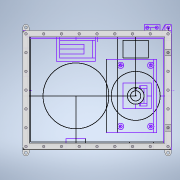
# Autodesk Inventor part: deadbolt enclosure walls
Saved by Autodesk Inventor 2022 (Build 260153000, 153)
## iProperties
Created: 2021-11-30
Part Number: deadbolt enclosure walls
Material: Generic
Document SubType Name: Modeling
Designer: a-dubs
Density: 1 g/cm^3
Appearance: Default
Author: a-dubs
Autodesk Inventor part; units mm, degrees
ref_plane "YZ Plane" through (0, 0, 0) normal (1, 0, 0) x (0, 1, 0)
sketch "Sketch1" plane through (0, 0, 0) normal (0, 1, 0) x (-1, 0, 0)
  line L0 (0, 0) -> (61, 0)
  circle A0 centre (0, 0) radius 33.6
  circle A1 centre (61, 0) radius 8.5
  line L1 (69.5, 0) -> (69.5, 7.5)
  line L2 (69.5, 7.5) -> (69.5, -7.5)
  line L3 (69.5, -7.5) -> (65, -7.5)
  line L4 (69.5, 7.5) -> (65, 7.5)
  line L5 (69.5, 7.5) -> (72.5, 7.5)
  line L6 (72.5, 7.5) -> (72.5, -7.5)
  line L7 (72.5, -7.5) -> (69.5, -7.5)
  line L8 (52.5, 0) -> (47.5, 0)
  line L9 (61, 8.5) -> (61, 13.5)
  line L10 (72.5, 0) -> (77.5, 0)
  line L11 (61, -8.5) -> (61, -13.5)
  line L12 (47.95, 13.05) -> (77.05, 13.05)
  line L13 (77.05, 13.05) -> (77.05, -13.05)
  line L14 (77.05, -13.05) -> (47.95, -13.05)
  line L15 (47.95, -13.05) -> (47.95, 13.05)
  line L16 (72.5, 7.5) -> (72.5, 10.5)
  line L17 (72.5, 10.5) -> (65, 10.5)
  line L18 (65, 10.5) -> (65, 7.5)
  line L19 (72.5, -7.5) -> (72.5, -10.5)
  line L20 (72.5, -10.5) -> (65, -10.5)
  line L21 (65, -10.5) -> (65, -7.5)
  line L22 (61, 0) -> (61, 60)
  line L23 (0, 0) -> (-42.65, 0)
  line L24 (-42.65, 0) -> (-47.65, 0)
  line L25 (0, 0) -> (0, -33.6)
  line L26 (0, 0) -> (42.65, 0)
  line L27 (42.65, 0) -> (42.65, 60)
  line L28 (42.65, 0) -> (42.65, -33.6)
  circle A2 centre (61, 0) radius 25
  line L29 (42.65, 25) -> (42.65, 31.2)
  line L30 (42.65, 31.2) -> (48.85, 31.2)
  line L31 (42.65, -25) -> (42.65, -31.2)
  line L32 (36, 0) -> (31, 0)
  line L33 (31, 0) -> (31, -31.2)
  line L34 (31, -31.2) -> (31, -37.4)
  line L35 (31, -37.4) -> (79.35, -37.4)
  line L36 (79.35, -37.4) -> (79.35, 31.2)
  line L37 (79.35, 31.2) -> (79.35, 37.4)
  line L38 (79.35, 37.4) -> (31, 37.4)
  line L39 (31, 37.4) -> (31, 0)
  line L40 (42.65, -33.6) -> (42.65, -37.4)
  circle A3 centre (61, 0) radius 5.25
  line L41 (86, 0) -> (91, 0)
  line L42 (91, 0) -> (97.4, 0)
  line L43 (-47.65, 0) -> (-47.65, 60)
  line L44 (-47.65, 60) -> (42.65, 60)
  line L45 (91, 0) -> (91, 60)
  line L46 (91, 60) -> (42.65, 60)
  line L47 (0, -33.6) -> (0, -43.6)
  line L48 (0, -43.6) -> (0, -48.6)
  line L49 (0, -48.6) -> (0, -55)
  line L50 (0, -55) -> (-54.05, -55)
  line L51 (0, -48.6) -> (-47.65, -48.6)
  line L52 (-47.65, -48.6) -> (-47.65, 0)
  line L53 (0, -55) -> (97.4, -55)
  line L54 (97.4, -55) -> (97.4, 0)
  line L55 (91, 0) -> (91, -48.6)
  line L56 (91, -48.6) -> (0, -48.6)
  line L57 (0, -48.6) -> (10, -48.6)
  line L58 (0, -48.6) -> (-10, -48.6)
  line L59 (10, -48.6) -> (10, -55)
  line L60 (-10, -48.6) -> (-10, -55)
  line L61 (10, -48.6) -> (10, -43.6)
  line L62 (10, -43.6) -> (-10, -43.6)
  line L63 (-10, -43.6) -> (-10, -49.0563)
  line L64 (65, 10.5) -> (66, 10.5)
  line L65 (66, 10.5) -> (66, 7.5)
  line L66 (65, -10.5) -> (66, -10.5)
  line L67 (66, -10.5) -> (66, -7.5)
  line L68 (-47.65, 0) -> (-54.05, 0)
  line L69 (42.65, 60) -> (42.65, 66.4)
  line L70 (-54.05, -55) -> (-54.05, 0)
  line L71 (-54.05, 66.4) -> (-54.05, 0)
  line L72 (42.65, 66.4) -> (-54.05, 66.4)
  line L73 (97.4, 0) -> (97.4, 66.4)
  line L74 (97.4, 66.4) -> (42.65, 66.4)
  line L75 (-47.65, 60) -> (-50.85, 60)
  line L76 (-50.85, 60) -> (-50.85, 63.2)
  circle A4 centre (-50.85, 63.2) radius 1.6
  line L77 (91, 60) -> (94.2, 60)
  line L78 (94.2, 60) -> (-50.85, 60)
  circle A5 centre (-32.7188, 63.2) radius 1.6
  circle A6 centre (-14.5875, 63.2) radius 1.6
  circle A7 centre (3.5437, 63.2) radius 1.6
  circle A8 centre (21.675, 63.2) radius 1.6
  circle A9 centre (39.8062, 63.2) radius 1.6
  circle A10 centre (57.9375, 63.2) radius 1.6
  circle A11 centre (76.0687, 63.2) radius 1.6
  circle A12 centre (94.2, 63.2) radius 1.6
  line L79 (-47.65, 60) -> (-47.65, 63.2)
  line L80 (-47.65, 63.2) -> (-47.65, -51.8)
  circle A13 centre (-50.85, 44.0333) radius 1.6
  circle A14 centre (-50.85, 24.8667) radius 1.6
  circle A15 centre (-50.85, 5.7) radius 1.6
  circle A16 centre (-50.85, -13.4667) radius 1.6
  circle A17 centre (-50.85, -32.6333) radius 1.6
  circle A18 centre (-50.85, -51.8) radius 1.6
  line L81 (-47.65, 60) -> (21.675, 60)
  line L82 (21.675, 60) -> (21.675, 55.1722)
  line L83 (-47.65, 5.7) -> (-45.15, 5.7)
  circle A19 centre (-32.7188, -51.8) radius 1.6
  circle A20 centre (-14.5875, -51.8) radius 1.6
  circle A21 centre (3.5437, -51.8) radius 1.6
  circle A22 centre (21.675, -51.8) radius 1.6
  circle A23 centre (39.8062, -51.8) radius 1.6
  circle A24 centre (57.9375, -51.8) radius 1.6
  circle A25 centre (76.0687, -51.8) radius 1.6
  circle A26 centre (94.2, -51.8) radius 1.6
  circle A27 centre (94.2, 44.0333) radius 1.6
  circle A28 centre (94.2, 24.8667) radius 1.6
  circle A29 centre (94.2, 5.7) radius 1.6
  circle A30 centre (94.2, -13.4667) radius 1.6
  circle A31 centre (94.2, -32.6333) radius 1.6
  line L84 (61, 60) -> (61, 56.8)
  line L85 (61, 56.8) -> (61, 38.8)
  line L86 (61, 56.8) -> (48.1, 56.8)
  line L87 (61, 56.8) -> (73.9, 56.8)
  line L88 (73.9, 56.8) -> (73.9, 38.8)
  line L89 (73.9, 38.8) -> (61, 38.8)
  line L90 (48.1, 56.8) -> (48.1, 38.8)
  line L91 (48.1, 38.8) -> (61, 38.8)
  line L92 (0, 60) -> (0, 56.8)
  line L93 (0, 56.8) -> (-16.65, 56.8)
  line L94 (-16.65, 56.8) -> (16.65, 56.8)
  line L95 (16.65, 56.8) -> (16.65, 38.6)
  line L96 (16.65, 38.6) -> (-16.65, 38.6)
  line L97 (-16.65, 38.6) -> (-16.65, 56.8)
  circle A32 centre (-50.85, 63.2) radius 1.4
  circle A33 centre (-32.7188, 63.2) radius 1.4
  circle A34 centre (-14.5875, 63.2) radius 1.4
  circle A35 centre (3.5437, 63.2) radius 1.4
  circle A36 centre (21.675, 63.2) radius 1.4
  circle A37 centre (39.8062, 63.2) radius 1.4
  circle A38 centre (57.9375, 63.2) radius 1.4
  circle A39 centre (76.0687, 63.2) radius 1.4
  circle A40 centre (94.2, 63.2) radius 1.4
  circle A41 centre (-50.85, -51.8) radius 1.4
  circle A42 centre (-32.7188, -51.8) radius 1.4
  circle A43 centre (-14.5875, -51.8) radius 1.4
  circle A44 centre (3.5437, -51.8) radius 1.4
  circle A45 centre (21.675, -51.8) radius 1.4
  circle A46 centre (39.8062, -51.8) radius 1.4
  circle A47 centre (57.9375, -51.8) radius 1.4
  circle A48 centre (76.0687, -51.8) radius 1.4
  circle A49 centre (94.2, -51.8) radius 1.4
  circle A50 centre (-50.85, 44.0333) radius 1.4
  circle A51 centre (-50.85, 24.8667) radius 1.4
  circle A52 centre (-50.85, 5.7) radius 1.4
  circle A53 centre (-50.85, -13.4667) radius 1.4
  circle A54 centre (-50.85, -32.6333) radius 1.4
  circle A55 centre (-50.85, -51.8) radius 1.4
  circle A56 centre (94.2, 63.2) radius 1.4
  circle A57 centre (94.2, 44.0333) radius 1.4
  circle A58 centre (94.2, 24.8667) radius 1.4
  circle A59 centre (94.2, 5.7) radius 1.4
  circle A60 centre (94.2, -13.4667) radius 1.4
  circle A61 centre (94.2, -32.6333) radius 1.4
  circle A62 centre (94.2, -51.8) radius 1.4
  line L98 (61, 8.5) -> (61, 6.7)
  line L99 (61, 6.7) -> (61.8, 6.7)
  line L100 (61, 6.7) -> (60.2, 6.7)
  line L101 (60.2, 6.7) -> (60.2, 8.4623)
  line L102 (61.8, 6.7) -> (61.8, 8.4623)
  line L103 (-16.65, 56.8) -> (-16.65, 60)
  line L104 (-16.65, 60) -> (-19.85, 60)
  line L105 (16.65, 38.6) -> (19.85, 38.6)
  line L106 (19.85, 38.6) -> (19.85, 35.4)
  line L107 (-19.85, 60) -> (19.85, 60)
  line L108 (19.85, 60) -> (19.85, 35.4)
  line L109 (19.85, 35.4) -> (-19.85, 35.4)
  line L110 (-19.85, 35.4) -> (-19.85, 60)
  line L111 (-16.65, 47.7) -> (8.35, 47.7)
  line L112 (16.65, 56.8) -> (19.85, 56.8)
  line L113 (16.65, 38.6) -> (19.85, 38.6)
  line L114 (8.35, 47.7) -> (8.35, 52.7)
  line L115 (8.35, 47.7) -> (8.35, 42.7)
  line L116 (8.35, 42.7) -> (-16.65, 42.7)
  line L117 (8.35, 52.7) -> (-16.65, 52.7)
  line L118 (79.35, -37.4) -> (82.55, -37.4)
  line L119 (82.55, -37.4) -> (82.55, 37.4)
  line L120 (82.55, 37.4) -> (79.35, 37.4)
  line L121 (48.85, 31.2) -> (45.65, 31.2)
  circle A63 centre (45.65, 31.2) radius 1.6
  circle A64 centre (45.65, 31.2) radius 1.4
  circle A65 centre (45.65, 31.2) radius 3.2
  circle A66 centre (76.35, 31.2) radius 1.6
  circle A67 centre (76.35, 31.2) radius 1.4
  circle A68 centre (76.35, 31.2) radius 3.2
  circle A69 centre (45.65, -31.2) radius 1.6
  circle A70 centre (45.65, -31.2) radius 1.4
  circle A71 centre (45.65, -31.2) radius 3.2
  circle A72 centre (76.35, -31.2) radius 3.2
  circle A73 centre (76.35, -31.2) radius 1.6
  circle A74 centre (76.35, -31.2) radius 1.4
  line L122 (91, -48.6) -> (92.6, -48.6)
  line L123 (92.6, -48.6) -> (92.6, -50.2)
  line L124 (-47.65, 60) -> (-49.25, 60)
  line L125 (-49.25, 60) -> (-49.25, 61.6)
  line L126 (-47.65, 60) -> (-46.05, 60)
  line L127 (-46.05, 60) -> (-46.05, 58.4)
  line L128 (91, -48.6) -> (89.4, -48.6)
  line L129 (89.4, -48.6) -> (89.4, -47)
  line L130 (89.4, -47) -> (-46.05, -47)
  line L131 (-46.05, -47) -> (-46.05, 58.4)
  line L132 (-46.05, 58.4) -> (89.4, 58.4)
  line L133 (89.4, 58.4) -> (89.4, -47)
  line L134 (-49.25, 61.6) -> (92.6, 61.6)
  line L135 (92.6, 61.6) -> (92.6, -50.2)
  line L136 (92.6, -50.2) -> (-49.25, -50.2)
  line L137 (-49.25, -50.2) -> (-49.25, 61.6)
  line L138 (76.0688, 66.4) -> (69.6688, 66.4)
  line L139 (76.0688, 66.4) -> (76.0688, 69.6)
  line L140 (76.0688, 69.6) -> (80.8688, 69.6)
  line L141 (76.0688, 69.6) -> (72.8688, 69.6)
  line L142 (80.8688, 69.6) -> (82.4688, 69.6)
  circle A75 centre (82.4688, 69.6) radius 1.6
  circle A76 centre (72.8688, 69.6) radius 1.6
  line L143 (69.6688, 66.4) -> (69.6688, 72.8)
  line L144 (76.0688, 66.4) -> (82.4688, 66.4)
  line L145 (82.4688, 66.4) -> (85.6688, 66.4)
  line L146 (85.6688, 66.4) -> (85.6688, 72.8)
  line L147 (85.6688, 72.8) -> (69.6688, 72.8)
  line L148 (57.9375, -51.8) -> (54.6375, -51.8)
  line L149 (54.6375, -51.8) -> (54.6375, -55)
  line L150 (54.6375, -51.8) -> (54.6375, -47)
  line L151 (76.0687, -51.8) -> (79.3687, -51.8)
  line L152 (79.3687, -51.8) -> (79.3688, -47)
  line L153 (79.3687, -51.8) -> (79.3688, -55)
  line L154 (-50.85, 44.0333) -> (-50.85, 48.8333)
  line L155 (-50.85, 24.8667) -> (-50.85, 20.0667)
  line L156 (-50.85, 48.8333) -> (-54.05, 48.8333)
  line L157 (-50.85, 48.8333) -> (-47.65, 48.8333)
  line L158 (-50.85, 20.0667) -> (-47.65, 20.0667)
  line L159 (-50.85, 20.0667) -> (-54.05, 20.0667)
  line L160 (94.2, 44.0333) -> (94.2, 47.4333)
  line L161 (94.2, 44.0333) -> (94.2, 40.6333)
  line L162 (94.2, -32.6333) -> (94.2, -29.2333)
  line L163 (94.2, -32.6333) -> (94.2, -36.0333)
  line L164 (94.2, -36.0333) -> (97.4, -36.0333)
  line L165 (94.2, -36.0333) -> (91, -36.0333)
  line L166 (94.2, -29.2333) -> (91, -29.2333)
  line L167 (94.2, -29.2333) -> (97.4, -29.2333)
  line L168 (94.2, 40.6333) -> (97.4, 40.6333)
  line L169 (94.2, 40.6333) -> (91, 40.6333)
  line L170 (94.2, 47.4333) -> (97.4, 47.4333)
  line L171 (94.2, 47.4333) -> (91, 47.4333)
  line L172 (97.4, 47.4333) -> (97.4, 55.4333)
  line L173 (94.2, 5.7) -> (97.4, 5.7)
  line L174 (97.4, 5.7) -> (97.4, 54.7)
  line L175 (97.4, 54.7) -> (97.4, 58.3)
  line L176 (97.4, 58.3) -> (91, 58.3)
  line L177 (97.4, 66.4) -> (97.4, 56.8)
  line L178 (97.4, 66.4) -> (87.8, 66.4)
  line L179 (87.8, 66.4) -> (87.8, 60)
  line L180 (97.4, 56.8) -> (91, 56.8)
  line L181 (94.2, 63.2) -> (94.2, 69.6)
  circle A77 centre (94.2, 69.6) radius 1.6
  line L182 (97.4, 66.4) -> (91, 66.4)
  line L183 (91, 66.4) -> (91, 72.8)
  line L184 (91, 72.8) -> (97.4, 72.8)
  line L185 (97.4, 72.8) -> (97.4, 66.4)
  line L186 (91, 72.8) -> (87.8, 66.4)
  line L187 (97.4, -55) -> (97.4, 66.4)
  line L188 (97.4, 66.4) -> (97.4, 5.7)
  line L189 (-50.85, 66.4) -> (-50.85, 63.2)
  point P0 (42.65, 37.4)
  point P1 (31, -12.9599)
  point P2 (31, 12.9599)
  point P3 (79.3688, -48.6)
  point P4 (54.6375, -48.6)
  dimension "d1" = 67.2
  dimension "d2" = 17
  dimension "d0" = 61
  dimension "d3" = 7.5
  dimension "d4" = 15
  dimension "d5" = 3
  dimension "d6" = 5
  dimension "d7" = 5
  dimension "d8" = 5
  dimension "d9" = 5
  dimension "d10" = 3
  dimension "d11" = 60
  dimension "d13" = 42.65
  dimension "d14" = 5
  dimension "d16" = 50
  dimension "d17" = 6.2
  dimension "d18" = 6.2
  dimension "d19" = 6.2
  dimension "d26" = 5
  dimension "d27" = 6.2
  dimension "d31" = 10.5
  dimension "d33" = 5
  dimension "d34" = 6.4
  dimension "d36" = 10
  dimension "d37" = 5
  dimension "d38" = 6.4
  dimension "d41" = 10
  dimension "d42" = 10
  dimension "d52" = 1
  dimension "d53" = 1
  dimension "d56" = 6.4
  dimension "d57" = 6.4
  dimension "d58" = 3.2
  dimension "d59" = 3.2
  dimension "d62" = 18.1313
  dimension "d67" = 115
  dimension "d70" = 19.1667
  dimension "d78" = 3.2
  dimension "d79" = 18
  dimension "d80" = 12.9
  dimension "d81" = 12.9
  dimension "d82" = 3.2
  dimension "d83" = 16.65
  dimension "d84" = 33.3
  dimension "d85" = 18.2
  dimension "d93" = 2.8
  dimension "d96" = 18.1313
  dimension "d99" = 115
  dimension "d104" = 19.1667
  dimension "d107" = 145.05
  dimension "d110" = 1.8
  dimension "d111" = 0.8
  dimension "d112" = 0.8
  dimension "d115" = 3.2
  dimension "d116" = 3.2
  dimension "d117" = 3.2
  dimension "d118" = 3.2
  dimension "d119" = 25
  dimension "d120" = 5
  dimension "d121" = 5
  dimension "d127" = 3.2
  dimension "d128" = 3.2
  dimension "d129" = 2.8
  dimension "d130" = 6.4
  dimension "d137" = 1.6
  dimension "d138" = 1.6
  constraints: 380 end point, 83 point on line, 75 centre point, 58 perpendicular, 33 vertical, 28 horizontal, 25 symmetric about line, 20 coincident, 16 parallel, 5 collinear, 5 midpoint, 2 point on circle, 1 horizontal alignment, 125 other
  measures "d0" distance of L0.start L0.end
  measures "d3" distance of L1.start L1.end
  measures "d4" distance of L1.end L2.end
  measures "d5" distance of L1.end L5.end
  measures "d6" distance of L8.start L8.end
  measures "d7" distance of L9.start L9.end
  measures "d8" distance of L10.start L10.end
  measures "d9" distance of L11.start L11.end
  measures "d10" distance of L5.end L16.end
  measures "d11" distance of L22.start L22.end
  measures "d13" distance of L23.start L23.end
  measures "d14" distance of L23.end L24.end
  measures "d16" diameter of A2
  measures "d17" distance of L29.start L29.end
  measures "d18" distance of L29.end L30.end
  measures "d19" distance of L31.start L31.end
  measures "d26" distance of L32.start L32.end
  measures "d27" distance of L33.end L34.end
  measures "d31" diameter of A3
  measures "d33" distance of L41.start L41.end
  measures "d34" distance of L41.end L42.end
  measures "d36" distance of L25.end L47.end
  measures "d37" distance of L47.end L48.end
  measures "d38" distance of L48.end L49.end
  measures "d41" distance of L48.end L57.end
  measures "d42" distance of L48.end L58.end
  measures "d52" distance of L17.end L64.end
  measures "d53" distance of L20.end L66.end
  measures "d56" distance of L24.end L68.end
  measures "d57" distance of L27.end L69.end
  measures "d58" distance of L43.end L75.end
  measures "d59" diameter of A4
  measures "d62" distance of A4.centre A5.centre
  measures "d67" distance of L79.end L80.end
  measures "d70" distance of A4.centre A13.centre
  measures "d78" distance of L22.end L84.end
  measures "d79" distance of L84.end L85.end
  measures "d80" distance of L84.end L86.end
  measures "d81" distance of L84.end L87.end
  measures "d82" distance of L92.start L92.end
  measures "d83" distance of L92.end L93.end
  measures "d84" distance of L93.end L94.end
  measures "d85" distance of L94.end L95.end
  measures "d93" diameter of A32
  measures "d96" distance of A32.centre A33.centre
  measures "d99" distance of A32.centre A41.centre
  measures "d104" distance of A32.centre L154.start
  measures "d107" distance of A32.centre L181.start
  measures "d110" distance of L9.start L98.end
  measures "d111" distance of L98.end L99.end
  measures "d112" distance of L98.end L100.end
  measures "d115" distance of L93.end L103.end
  measures "d116" distance of L103.end L104.end
  measures "d117" distance of L95.end L105.end
  measures "d118" distance of L105.end L106.end
  measures "d119" distance of L111.start L111.end
  measures "d120" distance of L111.end L114.end
  measures "d121" distance of L111.end L115.end
  measures "d127" distance of L121.start L121.end
  measures "d128" diameter of A63
  measures "d129" diameter of A64
  measures "d130" diameter of A65
  measures "d137" distance of L122.end L123.end
  measures "d138" distance of L43.end L124.end
extrude "Extrusion13" add sketch "Sketch1" along normal blind 50 contours L68 L137 L158 L43 | L52 L80 L136 L137 L68 | L56 L59 L136 L49 | L49 L136 L60 L51 | L51 L60 L136 L80 | A20 | A19 | A17 | A16 | L137 L136 L60 L50 L70 L68 | A15 | L68 L71 L159 L158 L137 | A21 | L136 L59 L53 L49 | L49 L50 L60 L136 | L56 L150 L136 L59 | L69 L134 L179 L46 | L44 L79 L134 L69 | L158 L137 L157 L43 | L56 L152 L136 L150 | A23 | A22 | L136 L150 L149 L53 L59 | A5 | A6 | A7 | A8 | A9 | L134 L125 L75 L76 A4 L189 L72 L69 | A10 | A11 | L69 L74 L179 L134 | L157 L137 L75 L43 | L158 L155 A14 L137 | L71 L156 L154 A13 L137 A14 L155 L159 | L75 L125 L134 L79 | L56 L122 L123 L136 L152 | L136 A24 L148 L150 | L179 L134 L135 L77 L46 | L157 L156 L71 L72 L189 A4 L76 L75 L137 | L137 A13 L154 L157 | A14 | L149 L148 A24 L136 A25 L151 L153 L53 | L152 L151 A25 L136 | L136 L123 L135 L165 L164 L54 L53 L153 L152 | A24 | L45 L169 L135 L42 | L42 L135 L166 L55 | L77 L135 L176 L45 | L179 L74 L73 L176 L135 L134 | A13 | L55 L165 L135 L122 | A25 | L135 A29 L173 L73 L42 | A30 | L42 L54 L167 L166 L135 | L45 L171 L135 L169 | L166 L135 L165 L55 | L176 L135 L180 L45 | L189 A32 L76 A4 | A4 L76 A32 L189 | A28 | L135 L169 L168 L73 L173 A29 | A29 | L45 L180 L135 L171 | L135 A27 L161 L169 | L166 L162 A31 L135 | L176 L73 L180 L135 | L189 L76 A32 | A32 L76 L189 | L164 L163 A31 L162 L167 L54 | L135 A31 L163 L165 | L171 L160 A27 L135 | L135 L180 L73 L170 L171 | A27 L160 A57 L161 | L161 A27 L160 L170 L73 L168 | A31 L162 A61 L163 | A27 L161 A57 L160 | A31 L163 A61 L162 | L160 L161 A57 | A57 L161 L160 | L162 L163 A61 | A61 L163 L162 | A12 | A18 | A26 | A33 | A34 | A35 | A36 | A37 | A38 | A39 | A40 | A41 | A42 | A43 | A44 | A45 | A46 | A47 | A48 | A49 | A50 | A51 | A52 | A53 | A54 | A58 | A59 | A60
extrude "Extrusion14" [suppressed]
extrude "Extrusion15" [suppressed]
extrude "Extrusion16" [suppressed]
extrude "feet" add sketch "Sketch1" against normal blind 6.4 contours L179 L134 L135 L77 L46 | L77 L135 L176 L45 | L179 L74 L73 L176 L135 L134 | L176 L135 L180 L45 | L176 L73 L180 L135 | A12 | A40
chamfer "Chamfer3" distance 6.4 angle 30 1 edges at (-94.2, 0, 56.8) measured on face at (-93.1333, -2.1333, 56.8)
chamfer "Chamfer4" distance 6.4 angle 30 1 edges at (-87.8, 0, 63.2) measured on face at (-87.8, -2.1333, 64.2667)
fillet "Fillet11" radius 3.2 2 edges at (-94.2, 0, 53.1051) (-84.1051, 0, 63.2)
extrude "Extrusion18" add sketch "Sketch1" along normal blind 6.4 from surface at -6.4 contours L183 L184 L185 L74
fillet "Fillet12" radius 3.2 2 edges at (-97.4, -3.2, 72.8) (-91, -3.2, 72.8)
ref_plane "Work Plane1" through (-21.675, 0, -55) normal (1, 0, 0) x (0, 0, -1)
ref_plane "Work Plane2" through (54.05, 50, 5.7) normal (0, 0, -1) x (-1, 0, 0)
mirror "Mirror1" about plane through (-21.675, 0, -55) normal (1, 0, 0) of "Fillet12", "Extrusion18"
mirror "Mirror2" about plane through (-21.675, 0, -55) normal (1, 0, 0) of "feet", "Chamfer3", "Chamfer4", "Fillet11"
mirror "Mirror3" about plane through (54.05, 50, 5.7) normal (0, 0, -1) of "feet", "Chamfer3", "Chamfer4", "Fillet11", "Mirror2"
mirror "Mirror4" about plane through (54.05, 50, 5.7) normal (0, 0, -1) of "Fillet12", "Extrusion18", "Mirror1"
fillet "Fillet13" radius 3.2 5 edges at (-97.4, 25, -55) (-97.4, 25, 66.4) (54.05, 25, 66.4) (54.05, 25, -55) (54.05, -3.2, -55)
extrude "m3 holes" cut sketch "Sketch1" against normal blind 6.4 from surface at 50 contours L189 L76 A32 | A32 L76 L189 | L160 L161 A57 | A57 L161 L160 | L162 L163 A61 | A61 L163 L162 | A33 | A34 | A35 | A36 | A37 | A38 | A39 | A40 | A41 | A42 | A43 | A44 | A45 | A46 | A47 | A48 | A49 | A50 | A51 | A52 | A53 | A54 | A58 | A59 | A60
extrude "led bar mount cutouts" cut sketch "Sketch1" against normal blind 6.4 from surface at 50 contours L45 L171 L135 L169 | L166 L135 L165 L55 | L135 A27 L161 L169 | L166 L162 A31 L135 | L164 L163 A31 L162 L167 L54 | L135 A31 L163 L165 | L171 L160 A27 L135 | A27 L160 A57 L161 | L161 A27 L160 L170 L73 L168 | A31 L162 A61 L163 | A27 L161 A57 L160 | A31 L163 A61 L162 | L160 L161 A57 | A57 L161 L160 | L162 L163 A61 | A61 L163 L162
extrude "Extrusion21" cut sketch "Sketch1" against normal blind 6.4 from surface at 43.6 contours L160 L161 A57 | A57 L161 L160 | L162 L163 A61 | A61 L163 L162
body "Solid3"
